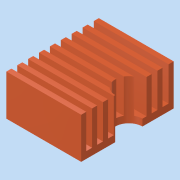
# Autodesk Inventor part: Heatsink
Saved by Autodesk Inventor 2017 (Build 210142000, 142)
## iProperties
Created: 2017-01-26
Part Number: Heatsink
Material: Aluminum 6061
Document SubType Name: Modeling
Designer: techn
Density: 2.7 g/cm^3
Appearance: Smooth - Light Orange
Author: techn
Autodesk Inventor part; units mm, degrees
ref_plane "YZ Plane" through (0, 0, 0) normal (1, 0, 0) x (0, 1, 0)
ref_plane "XZ Plane" through (0, 0, 0) normal (0, 1, 0) x (-1, 0, 0)
ref_plane "XY Plane" through (0, 0, 0) normal (0, 0, 1) x (1, 0, 0)
sketch "Sketch2" plane through (0, 0, 0) normal (0, 1, 0) x (-1, 0, 0)
  line L0 (0, 0) -> (22, 0)
  line L1 (22, 0) -> (22, -27.18)
  line L2 (22, -27.18) -> (0, -27.18)
  line L3 (0, -27.18) -> (0, 0)
  dimension "d0" = 27.18
  dimension "d1" = 22
  constraints: 8 end point, 2 parallel, 1 horizontal, 1 perpendicular
  measures "d0" distance of L2.end L0.start
  measures "d1" distance of L1.end L2.end
extrude "Extrusion1" add sketch "Sketch2" along normal blind 2
sketch "Sketch3" plane through (0, 2, 0) normal (0, 1, 0) x (1, 0, 0)
  line L0 (-22, 0) -> (0, 0) projected
  line L1 (0, 0) -> (0, 27.18) projected
  line L2 (0, 27.18) -> (-22, 27.18) projected
  line L3 (-22, 27.18) -> (-22, 0) projected
  line L4 (-22, 0) -> (0, 0) projected
  line L5 (0, 0) -> (0, 27.18) projected
  line L6 (-22, 0) -> (0, 0)
  line L7 (0, 0) -> (0, 1.5)
  line L8 (0, 1.5) -> (-22, 1.5)
  line L9 (-22, 1.5) -> (-22, 0)
  line L10 (-22, 3.2) -> (0, 3.2)
  line L11 (0, 3.2) -> (0, 4.7)
  line L12 (0, 4.7) -> (-22, 4.7)
  line L13 (-22, 4.7) -> (-22, 3.2)
  line L14 (-22, 6.4) -> (0, 6.4)
  line L15 (0, 6.4) -> (0, 7.9)
  line L16 (0, 7.9) -> (-22, 7.9)
  line L17 (-22, 7.9) -> (-22, 6.4)
  line L18 (-22, 9.6) -> (0, 9.6)
  line L19 (0, 9.6) -> (0, 11.1)
  line L20 (0, 11.1) -> (-22, 11.1)
  line L21 (-22, 11.1) -> (-22, 9.6)
  line L22 (-22, 12.8) -> (0, 12.8)
  line L23 (0, 12.8) -> (0, 14.3)
  line L24 (0, 14.3) -> (-22, 14.3)
  line L25 (-22, 14.3) -> (-22, 12.8)
  line L26 (-22, 16) -> (0, 16)
  line L27 (0, 16) -> (0, 17.5)
  line L28 (0, 17.5) -> (-22, 17.5)
  line L29 (-22, 17.5) -> (-22, 16)
  line L30 (-22, 19.2) -> (0, 19.2)
  line L31 (0, 19.2) -> (0, 20.7)
  line L32 (0, 20.7) -> (-22, 20.7)
  line L33 (-22, 20.7) -> (-22, 19.2)
  line L34 (-22, 22.4) -> (0, 22.4)
  line L35 (0, 22.4) -> (0, 23.9)
  line L36 (0, 23.9) -> (-22, 23.9)
  line L37 (-22, 23.9) -> (-22, 22.4)
  line L38 (-22, 27.18) -> (-22, 0) projected
  line L39 (0, 27.18) -> (-22, 27.18)
  line L40 (-22, 27.18) -> (-22, 25.68)
  line L41 (-22, 25.68) -> (0, 25.68)
  line L42 (0, 25.68) -> (0, 27.18)
  dimension "d4" = 1.5
  dimension "d7" = 3.2
  dimension "d12" = 1.5
  constraints: 72 end point, 4 parallel, 2 horizontal, 2 perpendicular, 2 point on line, 1 vertical, 56 other
  measures "d4" distance between parallel lines of L0 L8
  measures "d7" distance of L7.end L11.end
  measures "d12" distance of L40.end L39.end
extrude "Extrusion2" add sketch "Sketch3" along normal blind 10 contours L3 L8 L1 L0 | L3 L12 L1 L10 | L3 L16 L1 L14 | L3 L20 L1 L18 | L3 L24 L1 L22 | L3 L28 L1 L26 | L3 L32 L1 L30 | L3 L36 L1 L34 | L3 L2 L1 L41
sketch "Sketch4" plane through (0, 0, 0) normal (0, -1, 0) x (1, 0, 0)
  circle A0 centre (0, -14) radius 4
  line L0 (0, -27.18) -> (0, 0)
  dimension "d15" = 8
  dimension "d16" = 14
  constraints: 2 end point, 1 centre point
  measures "d15" diameter of A0
  measures "d16" distance of A0.centre L0.end
extrude "Extrusion3" cut sketch "Sketch4" against normal through all
body "Solid1"
